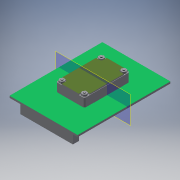
# Autodesk Inventor part: ADIS16448
Saved by Autodesk Inventor 2017 (Build 210142000, 142)
## iProperties
Created: 2016-12-19
Part Number: ADIS16448
Material: Generic
Document SubType Name: Modeling
Designer: Roksbot
Density: 1 g/cm^3
Appearance: Default
Author: Roksbot
Autodesk Inventor part; units mm, degrees
ref_plane "YZ Plane" through (0, 0, 0) normal (1, 0, 0) x (0, 1, 0)
ref_plane "XZ Plane" through (0, 0, 0) normal (0, 1, 0) x (-1, 0, 0)
ref_plane "XY Plane" through (0, 0, 0) normal (0, 0, 1) x (1, 0, 0)
sketch "Sketch1" plane through (0, 0, 0) normal (0, 1, 0) x (-1, 0, 0)
  line L0 (-28.4099, 38.7477) -> (28.4099, 38.7477)
  line L1 (28.4099, 38.7477) -> (28.4099, -38.7477)
  line L2 (28.4099, -38.7477) -> (-28.4099, -38.7477)
  line L3 (-28.4099, -38.7477) -> (-28.4099, 38.7477)
  line L4 (-28.4099, 38.7477) -> (28.4099, -38.7477) construction
  line L5 (28.4099, 38.7477) -> (-28.4099, -38.7477) construction
  point P0 (0, 0)
  dimension "d0" = 56.8198
  dimension "d1" = 77.4954
  constraints: 12 end point, 2 midpoint, 2 parallel, 1 horizontal, 1 perpendicular
  measures "d0" distance of L1.end L2.end
  measures "d1" distance of L0.end L1.end
extrude "Extrusion1" add sketch "Sketch1" along normal blind 1.524
sketch "Sketch2" plane through (0, 1.524, 0) normal (0, 1, 0) x (1, 0, 0)
  line L0 (11.8491, 21.3487) -> (7.4041, 21.3487) construction
  line L1 (-11.8491, 21.3487) -> (-11.8491, 16.2687) construction
  line L2 (-11.8491, -8.6233) -> (11.8491, -8.6233)
  line L3 (11.8491, -8.6233) -> (11.8491, 16.2687)
  line L4 (11.8491, 21.3487) -> (-11.8491, -8.6233) construction
  line L5 (-11.8491, 21.3487) -> (11.8491, -8.6233) construction
  line L6 (28.4099, 38.7477) -> (-28.4099, 38.7477) projected
  line L7 (-16.2941, 26.4287) -> (-7.4041, 26.4287)
  line L8 (-7.4041, 26.4287) -> (-7.4041, 19.4437)
  line L9 (-10.5791, 16.2687) -> (-16.2941, 16.2687)
  line L10 (-16.2941, 16.2687) -> (-16.2941, 26.4287) construction
  line L11 (-16.2941, 26.4287) -> (-7.4041, 16.2687) construction
  line L12 (-7.4041, 26.4287) -> (-16.2941, 16.2687) construction
  line L13 (16.2941, 26.4287) -> (7.4041, 26.4287)
  line L14 (7.4041, 26.4287) -> (7.4041, 21.3487)
  line L15 (10.5791, 16.2687) -> (11.8491, 16.2687)
  line L16 (16.2941, 16.2687) -> (16.2941, 26.4287)
  line L17 (16.2941, 26.4287) -> (7.4041, 16.2687) construction
  line L18 (7.4041, 26.4287) -> (16.2941, 16.2687) construction
  arc A0 (-10.5791, 16.2687) -> (-7.4041, 19.4437) centre (-10.5791, 19.4437) ccw
  arc A1 (7.4041, 19.4437) -> (10.5791, 16.2687) centre (10.5791, 19.4437) ccw
  line L19 (-11.8491, 16.2687) -> (-11.8491, -8.6233)
  line L20 (-7.4041, 21.3487) -> (-11.8491, 21.3487) construction
  line L21 (7.4041, 21.3487) -> (7.4041, 19.4437)
  line L22 (11.8491, 16.2687) -> (16.2941, 16.2687)
  line L23 (7.4041, 21.3487) -> (-7.4041, 21.3487)
  line L24 (11.8491, 16.2687) -> (11.8491, 21.3487) construction
  point P0 (0, 0)
  point P1 (0, 6.3627)
  point P2 (0, 6.3627)
  dimension "d4" = 23.6982
  dimension "d5" = 29.972
  dimension "d6" = 17.399
  dimension "d7" = 4.445
  dimension "d8" = 5.08
  dimension "d9" = 3.175
  constraints: 48 end point, 13 parallel, 9 perpendicular, 7 midpoint, 6 point on line, 6 tangent, 5 horizontal, 4 point on circle, 2 centre point, 1 collinear, 1 equal radius, 1 horizontal alignment, 1 vertical alignment
  measures "d4" distance of L0.start L1.start
  measures "d5" distance of L1.start L2.start
  measures "d6" distance between parallel lines of L6 L0
  measures "d7" distance between parallel lines of L1 L8
  measures "d8" distance between parallel lines of L0 L9
  measures "d9" radius of A0
extrude "Extrusion2" cut sketch "Sketch2" against normal through all contours L19 L9 A0 L8 L23 L21 A1 L15 L3 L2
ref_plane "Work Plane1" through (0, -0.9144, 0) normal (0, -1, 0) x (1, 0, 0)
sketch "Sketch3" plane through (0, -0.9144, 0) normal (0, -1, 0) x (1, 0, 0)
  line L0 (11.8491, 8.6233) -> (11.8491, -16.2687) projected
  line L1 (11.8491, -16.2687) -> (10.5791, -16.2687) projected
  arc A0 (10.5791, -16.2687) -> (7.4041, -19.4437) centre (10.5791, -19.4437) ccw projected
  line L2 (7.4041, -19.4437) -> (7.4041, -21.3487) projected
  line L3 (7.4041, -21.3487) -> (-7.4041, -21.3487) projected
  line L4 (-7.4041, -21.3487) -> (-7.4041, -19.4437) projected
  arc A1 (-7.4041, -19.4437) -> (-10.5791, -16.2687) centre (-10.5791, -19.4437) ccw projected
  line L5 (-10.5791, -16.2687) -> (-11.8491, -16.2687) projected
  line L6 (-11.8491, -16.2687) -> (-11.8491, 8.6233) projected
  line L7 (-11.8491, 8.6233) -> (11.8491, 8.6233) projected
  line L8 (28.4099, 38.7477) -> (-28.4099, 38.7477) projected
  line L9 (-28.4099, 38.7477) -> (-28.4099, -38.7477) projected
  line L10 (-28.4099, -38.7477) -> (28.4099, -38.7477) projected
  line L11 (28.4099, -38.7477) -> (28.4099, 38.7477) projected
  point P0 (0, 0)
extrude "Extrusion3" add sketch "Sketch3" against normal blind 2.54 contours L0 L1 A0 L2 L3 L4 A1 L5 L6 L7
sketch "Sketch4" plane through (0, 1.6256, 0) normal (0, 1, 0) x (1, 0, 0)
  line L0 (-11.8491, -16.4973) -> (11.8491, -16.4973)
  line L1 (11.8491, -16.4973) -> (11.8491, 21.3487)
  line L2 (11.8491, 21.3487) -> (-11.8491, 21.3487)
  line L3 (-11.8491, 21.3487) -> (-11.8491, -16.4973)
  line L4 (28.4099, 38.7477) -> (-28.4099, 38.7477) projected
  point P0 (0, 0)
  point P1 (-11.8491, -8.6233)
  point P2 (11.8491, 16.2687)
  point P3 (-7.4041, 21.3487)
  dimension "d15" = 37.846
  constraints: 8 end point, 2 parallel, 2 vertical alignment, 1 horizontal, 1 perpendicular, 1 point on line
  measures "d15" distance of L2.end L0.start
extrude "Extrusion4" add sketch "Sketch4" along normal blind 7.112
fillet "Fillet1" radius 1.27 10 edges at (11.8491, 5.1816, -21.3487) (-11.8491, 5.1816, -21.3487) (11.8491, 5.1816, 16.4973) (-11.8491, 5.1816, 16.4973) (11.8491, -0.4572, 8.6233) (-11.8491, -0.4572, 8.6233) (11.8491, -0.4572, -16.2687) (7.4041, -0.4572, -21.3487) (-7.4041, -0.4572, -21.3487) (-11.8491, -0.4572, -16.2687)
fillet "Fillet2" radius 0.508 14 edges at (11.4772, -0.9144, -15.8968) (10.5792, -0.9144, -16.2687) (8.334, -0.9144, -17.1986) (7.0322, -0.9144, -20.9768) (0, -0.9144, -21.3487) (-7.0322, -0.9144, -20.9768) (-10.5792, -0.9144, -16.2687) (-8.334, -0.9144, -17.1986) (-11.4772, -0.9144, -15.8968) (-11.8491, -0.9144, -3.8227) (-11.4772, -0.9144, 8.2514) (0, -0.9144, 8.6233) (11.4772, -0.9144, 8.2514) (11.8491, -0.9144, -3.8227)
sketch "Sketch5" plane through (0, 8.7376, 0) normal (0, 1, 0) x (1, 0, 0)
  circle A0 centre (-9.3726, 18.8722) radius 0.9525
  circle A1 centre (9.3726, 18.8722) radius 0.9525
  circle A2 centre (-9.3726, -14.0208) radius 0.9525
  circle A3 centre (9.3726, -14.0208) radius 0.9525
  line L0 (10.5791, 21.3487) -> (-10.5791, 21.3487) projected
  line L1 (-11.8491, 20.0787) -> (-11.8491, -15.2273) projected
  line L2 (-10.5791, -16.4973) -> (10.5791, -16.4973) projected
  line L3 (11.8491, -15.2273) -> (11.8491, 20.0787) projected
  point P0 (0, 0)
  dimension "d21" = 3.429
  dimension "d22" = 3.429
  dimension "d23" = 3.429
  dimension "d24" = 3.429
  dimension "d52" = 1.905
  constraints: 4 centre point, 3 equal radius, 2 horizontal alignment, 2 vertical alignment
  measures "d52" diameter of A0
extrude "Extrusion5" add sketch "Sketch5" along normal blind 2.032
thread "Thread1" size "100-102 UNM" class "2A" standard "ANSI Unified Screw Threads" full length
thread "Thread2" size "100-102 UNM" class "2A" standard "ANSI Unified Screw Threads" full length
thread "Thread3" size "100-102 UNM" class "2A" standard "ANSI Unified Screw Threads" full length
thread "Thread4" size "100-102 UNM" class "2A" standard "ANSI Unified Screw Threads" full length
sketch "Sketch6" plane through (0, 8.7376, 0) normal (0, 1, 0) x (1, 0, 0)
  circle A0 centre (-9.3726, -14.0208) radius 0.9525 projected
  circle A1 centre (-9.3726, 18.8722) radius 0.9525 projected
  circle A2 centre (9.3726, 18.8722) radius 0.9525 projected
  circle A3 centre (9.3726, -14.0208) radius 0.9525 projected
  arc A4 (-11.8491, -15.2273) -> (-10.5791, -16.4973) centre (-10.5791, -15.2273) ccw projected
  line L0 (-10.5791, -16.4973) -> (10.5791, -16.4973) projected
  arc A5 (10.5791, -16.4973) -> (11.8491, -15.2273) centre (10.5791, -15.2273) ccw projected
  line L1 (11.8491, -15.2273) -> (11.8491, 20.0787) projected
  arc A6 (11.8491, 20.0787) -> (10.5791, 21.3487) centre (10.5791, 20.0787) ccw projected
  line L2 (10.5791, 21.3487) -> (-10.5791, 21.3487) projected
  arc A7 (-10.5791, 21.3487) -> (-11.8491, 20.0787) centre (-10.5791, 20.0787) ccw projected
  line L3 (-11.8491, 20.0787) -> (-11.8491, -15.2273) projected
  line L4 (-10.5791, -16.4973) -> (10.5791, -16.4973) projected
  line L5 (-7.1501, 21.0947) -> (7.1501, 21.0947)
  line L6 (7.1501, -16.4973) -> (-7.1501, -16.4973)
  line L7 (11.5951, 16.6497) -> (11.5951, -11.7983)
  line L8 (-11.5951, -11.7983) -> (-11.5951, 16.6497)
  line L9 (-7.1501, -16.4973) -> (-7.1501, -11.7983)
  line L10 (-7.1501, 16.6497) -> (-7.1501, 21.0947)
  line L11 (-11.5951, 16.6497) -> (-7.1501, 16.6497)
  line L12 (7.1501, 16.6497) -> (11.5951, 16.6497)
  line L13 (7.1501, 21.0947) -> (7.1501, 16.6497)
  line L14 (7.1501, -11.7983) -> (7.1501, -16.4973)
  line L15 (11.5951, -11.7983) -> (7.1501, -11.7983)
  line L16 (-7.1501, -11.7983) -> (-11.5951, -11.7983)
  point P0 (0, 0)
  point P1 (-11.5951, 2.4257)
  point P2 (-11.8491, 2.4257)
  point P3 (-9.3726, 16.6497)
  point P4 (-7.1501, 18.8722)
  point P5 (7.1501, 18.8722)
  point P6 (0, 21.0947)
  point P7 (0, 21.3487)
  dimension "d49" = 4.445
  constraints: 24 end point, 10 parallel, 7 midpoint, 5 horizontal alignment, 4 perpendicular, 4 vertical alignment, 3 horizontal, 2 equal length, 1 point on line
  measures "d49" distance of L5.end L12.start
extrude "Extrusion6" add sketch "Sketch6" along normal blind 0.8636 contours L9 L16 L8 L11 L10 L5 L13 L12 L7 L15 L14 L0
fillet "Fillet3" radius 1.27 4 edges at (7.1501, 9.1694, 11.7983) (7.1501, 9.1694, -16.6497) (-7.1501, 9.1694, -16.6497) (-7.1501, 9.1694, 11.7983)
sketch "Sketch7" plane through (0, 8.7376, 0) normal (0, 1, 0) x (1, 0, 0)
  arc A0 (-7.1501, -13.0683) -> (-8.4201, -11.7983) centre (-8.4201, -13.0683) ccw projected
  line L0 (-8.4201, -11.7983) -> (-11.5951, -11.7983) projected
  line L1 (-11.5951, -11.7983) -> (-11.5951, 16.6497) projected
  line L2 (-11.5951, 16.6497) -> (-8.4201, 16.6497) projected
  arc A1 (-8.4201, 16.6497) -> (-7.1501, 17.9197) centre (-8.4201, 17.9197) ccw projected
  line L3 (-7.1501, 17.9197) -> (-7.1501, 21.0947) projected
  line L4 (-7.1501, 21.0947) -> (7.1501, 21.0947) projected
  line L5 (7.1501, 21.0947) -> (7.1501, 17.9197) projected
  arc A2 (7.1501, 17.9197) -> (8.4201, 16.6497) centre (8.4201, 17.9197) ccw projected
  line L6 (8.4201, 16.6497) -> (11.5951, 16.6497) projected
  line L7 (11.5951, 16.6497) -> (11.5951, -11.7983) projected
  line L8 (11.5951, -11.7983) -> (8.4201, -11.7983) projected
  arc A3 (8.4201, -11.7983) -> (7.1501, -13.0683) centre (8.4201, -13.0683) ccw projected
  line L9 (7.1501, -13.0683) -> (7.1501, -16.4973) projected
  line L10 (7.1501, -16.4973) -> (10.5791, -16.4973) projected
  arc A4 (10.5791, -16.4973) -> (11.8491, -15.2273) centre (10.5791, -15.2273) ccw projected
  line L11 (11.8491, -15.2273) -> (11.8491, 20.0787) projected
  arc A5 (11.8491, 20.0787) -> (10.5791, 21.3487) centre (10.5791, 20.0787) ccw projected
  line L12 (10.5791, 21.3487) -> (-10.5791, 21.3487) projected
  arc A6 (-10.5791, 21.3487) -> (-11.8491, 20.0787) centre (-10.5791, 20.0787) ccw projected
  line L13 (-11.8491, 20.0787) -> (-11.8491, -15.2273) projected
  arc A7 (-11.8491, -15.2273) -> (-10.5791, -16.4973) centre (-10.5791, -15.2273) ccw projected
  line L14 (-10.5791, -16.4973) -> (-7.1501, -16.4973) projected
  line L15 (-7.1501, -16.4973) -> (-7.1501, -13.0683) projected
  circle A8 centre (9.3726, -14.0208) radius 0.9525 projected
  circle A9 centre (9.3726, 18.8722) radius 0.9525 projected
  circle A10 centre (-9.3726, 18.8722) radius 0.9525 projected
  circle A11 centre (-9.3726, -14.0208) radius 0.9525 projected
  line L16 (-11.231, 20.103) -> (-9.2359, 21.097)
  line L17 (-9.2359, 21.097) -> (-7.3775, 19.8662)
  line L18 (-7.3775, 19.8662) -> (-7.5142, 17.6414)
  line L19 (-7.5142, 17.6414) -> (-9.5093, 16.6474)
  line L20 (-9.5093, 16.6474) -> (-11.3677, 17.8782)
  line L21 (-11.3677, 17.8782) -> (-11.231, 20.103)
  line L22 (8.0127, 17.106) -> (7.1631, 19.1668)
  line L23 (7.1631, 19.1668) -> (8.523, 20.933)
  line L24 (8.523, 20.933) -> (10.7325, 20.6384)
  line L25 (10.7325, 20.6384) -> (11.5821, 18.5776)
  line L26 (11.5821, 18.5776) -> (10.2222, 16.8114)
  line L27 (10.2222, 16.8114) -> (8.0127, 17.106)
  circle A12 centre (9.3726, -14.0208) radius 0.9525 projected
  line L28 (8.1576, -15.8896) -> (7.1467, -13.903)
  line L29 (7.1467, -13.903) -> (8.3617, -12.0342)
  line L30 (8.3617, -12.0342) -> (10.5876, -12.152)
  line L31 (10.5876, -12.152) -> (11.5985, -14.1386)
  line L32 (11.5985, -14.1386) -> (10.3835, -16.0074)
  line L33 (10.3835, -16.0074) -> (8.1576, -15.8896)
  circle A13 centre (-9.3726, -14.0208) radius 0.9525 projected
  line L34 (-11.6016, -14.0223) -> (-10.4884, -12.0912)
  line L35 (-10.4884, -12.0912) -> (-8.2594, -12.0896)
  line L36 (-8.2594, -12.0896) -> (-7.1436, -14.0193)
  line L37 (-7.1436, -14.0193) -> (-8.2568, -15.9504)
  line L38 (-8.2568, -15.9504) -> (-10.4858, -15.952)
  line L39 (-10.4858, -15.952) -> (-11.6016, -14.0223)
  point P0 (0, 0)
  dimension "d45" = 3.8608
  constraints: 48 end point, 4 coincident, 3 equal length, 52 other
  measures "d45" distance between parallel lines of L18 L21
extrude "Extrusion7" add sketch "Sketch7" along normal blind 1.4732 contours L20 L21 L16 L17 L18 L19 | L36 L37 L15 | L15 L37 L38 L39 L34 L35 L36 | L28 L29 L9 | L9 L29 L30 L31 L32 L33 L28 | L22 L23 L24 L25 L26 L27
sketch "Sketch8" plane through (0, 0, 0) normal (0, -1, 0) x (1, 0, 0)
  arc A0 (-7.4041, -19.4437) -> (-10.5791, -16.2687) centre (-10.5791, -19.4437) ccw projected
  arc A1 (-11.8491, -14.9987) -> (-10.5791, -16.2687) centre (-10.5791, -14.9987) ccw projected
  line L0 (-11.8491, -14.9987) -> (-11.8491, 7.3533) projected
  arc A2 (-10.5791, 8.6233) -> (-11.8491, 7.3533) centre (-10.5791, 7.3533) ccw projected
  line L1 (-10.5791, 8.6233) -> (10.5791, 8.6233) projected
  arc A3 (11.8491, 7.3533) -> (10.5791, 8.6233) centre (10.5791, 7.3533) ccw projected
  line L2 (11.8491, 7.3533) -> (11.8491, -14.9987) projected
  arc A4 (10.5791, -16.2687) -> (11.8491, -14.9987) centre (10.5791, -14.9987) ccw projected
  arc A5 (10.5791, -16.2687) -> (7.4041, -19.4437) centre (10.5791, -19.4437) ccw projected
  arc A6 (6.1341, -21.3487) -> (7.4041, -20.0787) centre (6.1341, -20.0787) ccw projected
  line L3 (6.1341, -21.3487) -> (-6.1341, -21.3487) projected
  arc A7 (-7.4041, -20.0787) -> (-6.1341, -21.3487) centre (-6.1341, -20.0787) ccw projected
  line L4 (28.4099, 38.7477) -> (-28.4099, 38.7477) projected
  line L5 (-28.4099, 38.7477) -> (-28.4099, -38.7477) projected
  line L6 (-28.4099, -38.7477) -> (28.4099, -38.7477) projected
  line L7 (28.4099, -38.7477) -> (28.4099, 38.7477) projected
  circle A8 centre (-9.3726, 14.0208) radius 0.9525 projected
  circle A9 centre (9.3726, 14.0208) radius 0.9525 projected
  circle A10 centre (9.3726, -18.8722) radius 0.9525 projected
  circle A11 centre (-9.3726, -18.8722) radius 0.9525 projected
  line L8 (7.4041, -19.4437) -> (7.4041, -20.0787) projected
  line L9 (-7.4041, -20.0787) -> (-7.4041, -19.4437) projected
  circle A12 centre (-9.3726, 14.0208) radius 1.9304
  circle A13 centre (9.3726, 14.0208) radius 1.9304
  circle A14 centre (9.3726, -18.8722) radius 1.9304
  circle A15 centre (-9.3726, -18.8722) radius 1.9304
  point P0 (0, 0)
  dimension "d53" = 3.8608
  constraints: 4 centre point, 4 coincident, 3 equal radius
  measures "d53" diameter of A12
extrude "Extrusion8" add sketch "Sketch8" along normal up to surface (0.9144 mm away) contours A15 A0 | A0 A15 | A14 A5 | A5 A14 | A8 | A9 | A10 | A11 | A12 | A13
fillet "Fillet4" radius 1.27 4 edges at (-11.303, -0.9144, 14.0208) (7.4422, -0.9144, 14.0208) (7.4422, -0.9144, -18.8722) (-11.303, -0.9144, -18.8722)
sketch "Sketch9" plane through (0, 0, 0) normal (0, -1, 0) x (1, 0, 0)
  line L0 (21.9075, 31.1277) -> (-21.9075, 31.1277)
  line L1 (-21.9075, 31.1277) -> (-21.9075, 36.2077)
  line L2 (-21.9075, 36.2077) -> (21.9075, 36.2077)
  line L3 (21.9075, 36.2077) -> (21.9075, 31.1277)
  line L4 (21.9075, 31.1277) -> (-21.9075, 36.2077) construction
  line L5 (-21.9075, 31.1277) -> (21.9075, 36.2077) construction
  line L6 (28.4099, 38.7477) -> (-28.4099, 38.7477) projected
  point P0 (0, 0)
  point P1 (0, 33.6677)
  point P2 (0, 33.6677)
  point P3 (0, 38.7477)
  dimension "d57" = 5.08
  dimension "d58" = 43.815
  dimension "d59" = 2.54
  constraints: 12 end point, 4 midpoint, 2 parallel, 1 horizontal, 1 perpendicular, 1 vertical alignment
  measures "d57" distance of L2.end L0.start
  measures "d58" distance of L1.end L2.end
  measures "d59" distance between parallel lines of L2 L6
extrude "Extrusion9" add sketch "Sketch9" along normal blind 9.779
ref_plane "Work Plane2" through (7.4041, 1.524, -2.4257) normal (0, 0, -1) x (-1, 0, 0)
sketch "Sketch10" plane through (0, 0, 0) normal (0, -1, 0) x (1, 0, 0)
  circle A0 centre (24.6253, -35.0647) radius 1.5875
  circle A1 centre (-24.6253, -35.0647) radius 1.5875
  line L0 (-28.4099, -38.7477) -> (28.4099, -38.7477) projected
  line L1 (-28.4099, 38.7477) -> (-28.4099, -38.7477) projected
  line L2 (28.4099, -38.7477) -> (28.4099, 38.7477) projected
  point P0 (0, 0)
  dimension "d62" = 3.175
  dimension "d63" = 2.0955
  dimension "d64" = 2.1971
  dimension "d65" = 2.1971
  constraints: 2 centre point, 1 equal radius, 1 horizontal alignment
  measures "d62" diameter of A1
  measures "d63" distance edge to line of A1 L0
  measures "d64" distance edge to line of A1 L1
  measures "d65" distance edge to line of A0 L2
extrude "Extrusion10" cut sketch "Sketch10" against normal through all
equation "\"d22\" = d21"
equation "\"d23\" = d22"
equation "\"d24\" = d21"
equation "\"d65\" = d64"
body "Solid1"
